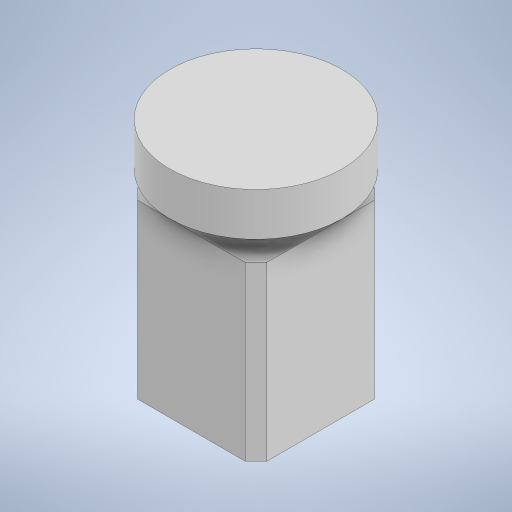
# Autodesk Inventor part: Motor
Saved by Autodesk Inventor 2023 (Build 270158030, 158C)
## iProperties
Created: 2023-02-13
Part Number: Motor
Material: Generic
Document SubType Name: Modeling
Designer: jeremyy
Density: 1 g/cm^3
Appearance: Default
Author: jeremyy
Autodesk Inventor part; units mm, degrees
ref_plane "YZ Plane" through (0, 0, 0) normal (1, 0, 0) x (0, 1, 0)
ref_plane "XZ Plane" through (0, 0, 0) normal (0, 1, 0) x (-1, 0, 0)
ref_plane "XY Plane" through (0, 0, 0) normal (0, 0, 1) x (1, 0, 0)
sketch "Sketch1" plane through (0, 0, 0) normal (0, 1, 0) x (-1, 0, 0)
  line L0 (6.35, 0) -> (69.85, 0)
  line L1 (76.2, -6.35) -> (76.2, -69.85)
  line L2 (69.85, -76.2) -> (6.35, -76.2)
  line L3 (0, -69.85) -> (0, -6.35)
  line L4 (69.85, 0) -> (76.2, -6.35)
  line L5 (76.2, -69.85) -> (69.85, -76.2)
  line L6 (6.35, 0) -> (0, -6.35)
  line L7 (6.35, -76.2) -> (0, -69.85)
  point P0 (0, 0)
  point P1 (76.2, -76.2)
  point P2 (76.2, 0)
  point P3 (0, -76.2)
  dimension "d2" = 76.2
  dimension "d3" = 76.2
  dimension "d4" = 6.35
  dimension "d5" = 6.35
  dimension "d6" = 6.35
  dimension "d7" = 6.35
  dimension "d8" = 6.35
  dimension "d9" = 6.35
  dimension "d10" = 6.35
  dimension "d11" = 6.35
  constraints: 16 end point, 8 point on line, 2 parallel, 1 horizontal, 1 perpendicular
  measures "d2" distance between parallel lines of L2 L0
  measures "d3" distance between parallel lines of L3 L1
  measures "d4" distance of L0.end point (76.2, 0)
  measures "d5" distance of L1.start point (76.2, 0)
  measures "d6" distance of L1.end point (76.2, -76.2)
  measures "d7" distance of L2.start point (76.2, -76.2)
  measures "d8" distance of L0.start point (0, 0)
  measures "d9" distance of L3.end point (0, 0)
  measures "d10" distance of L2.end point (0, -76.2)
  measures "d11" distance of L3.start point (0, -76.2)
extrude "Extrusion1" add sketch "Sketch1" along normal blind 101.6
sketch "Sketch2" plane through (0, 101.6, 0) normal (0, 1, 0) x (1, 0, 0)
  circle A0 centre (-38.1, 38.1) radius 19.05
  line L0 (-69.85, 0) -> (-6.35, 0) projected
  line L1 (0, 6.35) -> (0, 69.85) projected
  point P0 (0, 0)
  dimension "d14" = 38.1
  dimension "d15" = 38.1
  dimension "d16" = 38.1
  constraints: 1 centre point
  measures "d14" diameter of A0
  measures "d15" distance from line of L0 A0.centre
  measures "d16" distance from line of L1 A0.centre
extrude "Extrusion2" add sketch "Sketch2" along normal blind 12.7
sketch "Sketch3" plane through (-38.1, 114.3, -38.1) normal (0, 1, 0) x (1, 0, 0)
  circle A0 centre (0, 0) radius 50.8
  point P0 (38.1, -38.1)
  dimension "d19" = 101.6
  constraints: 1 centre point
  measures "d19" diameter of A0
extrude "Extrusion3" add sketch "Sketch3" along normal blind 25.4
body "Solid1"
